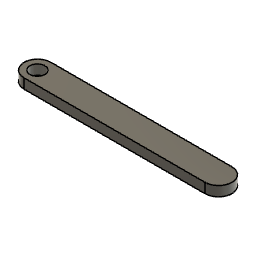
Magnet_Storage_Latch (Autodesk Fusion 360 design; units mm, degrees)
Autodesk Fusion 360 part; units mm, degrees
sketch "Sketch1" plane through (0, 0, 0) normal (0, 1, 0) x (1, 0, 0)
  circle A0 centre (0, 0) radius 1.55
  circle A1 centre (0, 0) radius 2.75
  line L0 (0, 2.75) -> (37, 2.75)
  line L1 (29.0028, 0) -> (29.0028, 0)
  line L2 (37, -2.75) -> (0, -2.75)
  arc A2 (39.75, 0) -> (37, 2.75) centre (37, 0) ccw
  arc A3 (37, -2.75) -> (39.75, 0) centre (37, 0) ccw
  dimension "d1" = 3.1
  dimension "d3" = 5.5
  dimension "d4" = 2.75
  dimension "d6" = 37
  constraint coincident A0.centre A1.centre
  constraint concentric A0 A1
  constraint coincident A1 L0.start
  constraint horizontal L0
  constraint coincident A1 L2.end
  constraint tangent A1 L2
  constraint tangent A1 L0
  constraint horizontal L2
  constraint tangent L0 A2
  constraint tangent L2 A3
  constraint equal A2 A3
  constraint tangent A2 A3
  measures "d1" diameter of A0
  measures "d3" diameter of A1
  measures "d4" radius of A2
  measures "d6" distance of A0.centre A2.centre
extrude "Extrude1" add sketch "Sketch1" along normal blind 2
equation "d6 = 40 mm - d4 - 0.25 mm"
